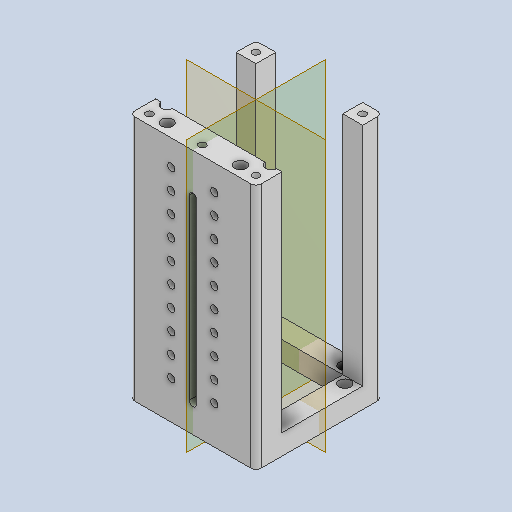
# Autodesk Inventor part: 00_Linear_Stage_NEMA11_Mount
Saved by Autodesk Inventor 2023 (Build 270158000, 158)
## iProperties
Created: 2022-02-11
Part Number: 00_Linear_Stage_NEMA11_Mount
Material: Generic
Document SubType Name: Modeling
Designer: wanghaoran
Density: 1 g/cm^3
Appearance: Default
Author: wanghaoran
Autodesk Inventor part; units mm, degrees
ref_plane "YZ Plane" through (0, 0, 0) normal (1, 0, 0) x (0, 1, 0)
ref_plane "XZ Plane" through (0, 0, 0) normal (0, 1, 0) x (-1, 0, 0)
ref_plane "XY Plane" through (0, 0, 0) normal (0, 0, 1) x (1, 0, 0)
sketch "Sketch1" plane through (0, 0, 0) normal (0, 1, 0) x (-1, 0, 0)
  line L0 (0, 0) -> (49.8, 0)
  line L1 (49.8, 0) -> (49.8, -49.8)
  line L2 (49.8, -49.8) -> (0, -49.8)
  line L3 (0, -49.8) -> (0, 0)
  line L4 (7.8, -7.8) -> (42, -7.8)
  line L5 (42, -7.8) -> (42, -42)
  line L6 (42, -42) -> (7.8, -42)
  line L7 (7.8, -42) -> (7.8, -7.8)
  dimension "d0" = 49.8
  dimension "d1" = 49.8
  dimension "d2" = 7.8
  constraints: 16 end point, 4 parallel, 2 perpendicular, 1 horizontal, 3 other
  measures "d0" distance of L1.end L2.end
  measures "d1" distance of L0.end L1.end
  measures "d2" distance between parallel lines of L3 L7
extrude "Extrusion1" add sketch "Sketch1" along normal blind 8
sketch "Sketch3" plane through (0, 0, 0) normal (0, -1, 0) x (1, 0, 0)
  line L0 (-49.8, 0) -> (0, 0) projected
  line L1 (-49.8, -49.8) -> (-49.8, 0) projected
  line L2 (0, 0) -> (-49.8, 0)
  line L3 (-49.8, 0) -> (-49.8, -10.23)
  line L4 (-49.8, -10.23) -> (0, -10.23)
  line L5 (0, -10.23) -> (0, 0)
  line L6 (-7.8, -42) -> (-7.8, -7.8) projected
  line L7 (0, -49.8) -> (-7.8, -49.8)
  line L8 (-7.8, -49.8) -> (-7.8, -42)
  line L9 (-7.8, -42) -> (0, -42)
  line L10 (0, -42) -> (0, -49.8)
  line L11 (0, -49.8) -> (-49.8, -49.8) projected
  line L12 (-42, -7.8) -> (-42, -42) projected
  line L13 (-49.8, -49.8) -> (-42, -49.8)
  line L14 (-42, -49.8) -> (-42, -42)
  line L15 (-42, -42) -> (-49.8, -42)
  line L16 (-49.8, -42) -> (-49.8, -49.8)
  dimension "d6" = 10.23
  constraints: 24 end point, 6 parallel, 3 horizontal, 3 perpendicular, 1 point on line
  measures "d6" distance of L3.end L2.end
extrude "Extrusion2" add sketch "Sketch3" against normal blind 97 contours L0 L5 L4 L1 | L15 L14 L11 L1 | L9 L10 L7 L8
sketch "Sketch4" plane through (-49.8, 0, 0) normal (0, 0, 1) x (1, 0, 0)
  line L0 (23.45, 81) -> (26.35, 81)
  line L1 (26.35, 81) -> (26.35, 11)
  line L2 (26.35, 11) -> (23.45, 11)
  line L3 (23.45, 11) -> (23.45, 81)
  line L4 (49.8, 0) -> (49.8, 97) projected
  line L5 (0, 0) -> (49.8, 0) projected
  circle A0 centre (24.9, 81) radius 1.45
  circle A1 centre (24.9, 11) radius 1.45
  circle A2 centre (16.4, 87) radius 1.45
  circle A3 centre (33.4, 87) radius 1.45
  line L6 (0, 97) -> (49.8, 97) projected
  circle A4 centre (16.4, 79) radius 1.45
  circle A5 centre (33.4, 79) radius 1.45
  circle A6 centre (16.4, 71) radius 1.45
  circle A7 centre (33.4, 71) radius 1.45
  circle A8 centre (16.4, 63) radius 1.45
  circle A9 centre (33.4, 63) radius 1.45
  circle A10 centre (16.4, 55) radius 1.45
  circle A11 centre (33.4, 55) radius 1.45
  circle A12 centre (16.4, 47) radius 1.45
  circle A13 centre (33.4, 47) radius 1.45
  circle A14 centre (16.4, 39) radius 1.45
  circle A15 centre (33.4, 39) radius 1.45
  circle A16 centre (16.4, 31) radius 1.45
  circle A17 centre (33.4, 31) radius 1.45
  circle A18 centre (16.4, 23) radius 1.45
  circle A19 centre (33.4, 23) radius 1.45
  circle A20 centre (16.4, 15) radius 1.45
  circle A21 centre (33.4, 15) radius 1.45
  point P0 (32.35, 97)
  point P1 (34.45, 97)
  dimension "d9" = 2.9
  dimension "d10" = 70
  dimension "d11" = 23.45
  dimension "d12" = 11
  dimension "d15" = 2.9
  dimension "d16" = 7.05
  dimension "d17" = 2.9
  dimension "d18" = 7.05
  dimension "d19" = 10
  dimension "d20" = 10
  dimension "d23" = 8
  dimension "d52" = 8
  constraints: 20 centre point, 8 end point, 2 midpoint, 2 parallel, 2 vertical, 1 horizontal, 1 perpendicular, 42 other
  measures "d9" distance of L1.end L2.end
  measures "d10" distance of L0.end L1.end
  measures "d11" distance between parallel lines of L4 L1
  measures "d12" distance between parallel lines of L5 L2
  measures "d15" diameter of A2
  measures "d16" distance from line of L3 A2.centre
  measures "d17" diameter of A3
  measures "d18" distance from line of A3.centre L1
  measures "d19" distance from line of L6 A2.centre
  measures "d20" distance from line of L6 A3.centre
  measures "d23" distance of A2.centre A4.centre
  measures "d52" distance of A14.centre A16.centre
extrude "Extrusion3" cut sketch "Sketch4" against normal through all
sketch "Sketch5" plane through (0, 97, 0) normal (0, 1, 0) x (1, 0, 0)
  circle A0 centre (-45.9, 45.9) radius 1.4
  circle A1 centre (-3.9, 45.9) radius 1.4
  line L0 (-49.8, 49.8) -> (-49.8, 0) projected
  line L1 (-49.8, 24.9) -> (-42, 24.9)
  line L2 (-42, 10.23) -> (-42, 42) projected
  circle A2 centre (-45.9, 3.9) radius 1.4
  circle A3 centre (-3.9, 3.9) radius 1.4
  point P0 (0, 0)
  dimension "d28" = 2.8
  dimension "d29" = 2.8
  constraints: 4 centre point, 2 end point, 2 symmetric about line, 1 horizontal, 1 midpoint, 1 point on line, 2 other
  measures "d28" diameter of A0
  measures "d29" diameter of A1
extrude "Extrusion4" cut sketch "Sketch5" against normal blind 20
sketch "Sketch6" plane through (0, 0, 0) normal (0, -1, 0) x (1, 0, 0)
  line L0 (-49.8, 0) -> (0, 0) projected
  circle A0 centre (-24.9, -3.7) radius 1.4
  line L1 (-49.8, -49.8) -> (-49.8, 0) projected
  dimension "d37" = 2.8
  dimension "d38" = 3.7
  dimension "d39" = 24.9
  constraints: 1 centre point
  measures "d37" diameter of A0
  measures "d38" distance from line of L0 A0.centre
  measures "d39" distance from line of L1 A0.centre
extrude "Extrusion5" cut sketch "Sketch6" against normal blind 10
fillet "Fillet1" radius 2 4 edges at (0, 48.5, 0) (0, 48.5, -49.8) (-49.8, 48.5, -49.8) (-49.8, 48.5, 0)
sketch "Sketch7" plane through (0, 97, 0) normal (0, 1, 0) x (1, 0, 0)
  circle A0 centre (-24.9, 3.7) radius 1.4 projected
  circle A1 centre (-24.9, 3.7) radius 1.4
  point P0 (0, 0)
  constraints: 1 centre point, 1 coincident
extrude "Extrusion6" cut sketch "Sketch7" against normal blind 10
ref_plane "Arbeitsebene1" through (-24.9, 8, -10.23) normal (-1, 0, 0) x (0, 0, 1)
ref_plane "Arbeitsebene2" through (-47.8, 0, -24.9) normal (0, 0, 1) x (1, 0, 0)
sketch "Skizze8" plane through (0, 0, 0) normal (0, -1, 0) x (1, 0, 0)
  line L0 (-49.9, -29.9) -> (-49.9, -47.9) projected
  arc A0 (-49.9, -47.9) -> (-47.9, -49.9) centre (-47.9, -47.9) ccw projected
  line L1 (-30.0511, -49.9) -> (-47.9, -49.9) projected
  line L2 (-30.0511, -49.9) -> (-30.0509, -49.1742) projected
  arc A1 (-30.0509, -49.1742) -> (-30.2806, -48.8498) centre (-30.3999, -49.1778) ccw projected
  arc A2 (-31.9947, -46.7407) -> (-30.2806, -48.8498) centre (-29.84, -46.7407) ccw projected
  line L3 (-31.9947, -46.7407) -> (-31.9947, -46.6009) projected
  arc A3 (-29.8434, -44.4498) -> (-31.9947, -46.6009) centre (-29.8435, -46.6009) ccw projected
  line L4 (-29.8434, -44.4498) -> (-19.9598, -44.4503) projected
  arc A4 (-17.81, -46.6004) -> (-19.9598, -44.4503) centre (-19.96, -46.6003) ccw projected
  line L5 (-17.81, -46.6004) -> (-17.81, -46.7408) projected
  arc A5 (-19.52, -48.8451) -> (-17.81, -46.7408) centre (-19.9599, -46.7406) ccw projected
  arc A6 (-19.52, -48.8451) -> (-19.7498, -49.1739) centre (-19.3996, -49.1739) ccw projected
  line L6 (-19.7498, -49.1739) -> (-19.7495, -49.9) projected
  line L7 (-1.9, -49.9) -> (-19.7495, -49.9) projected
  arc A7 (-1.9, -49.9) -> (0.1, -47.9) centre (-1.9, -47.9) ccw projected
  line L8 (0.1, -47.9) -> (0.1, -30.0511) projected
  line L9 (0.1, -30.0511) -> (-0.6258, -30.0509) projected
  arc A8 (-0.6258, -30.0509) -> (-0.9502, -30.2806) centre (-0.6222, -30.3999) ccw projected
  arc A9 (-3.0593, -31.9947) -> (-0.9502, -30.2806) centre (-3.0593, -29.84) ccw projected
  line L10 (-3.0593, -31.9947) -> (-3.1991, -31.9947) projected
  arc A10 (-5.3502, -29.8434) -> (-3.1991, -31.9947) centre (-3.1991, -29.8435) ccw projected
  line L11 (-5.3502, -29.8434) -> (-5.3497, -19.9598) projected
  arc A11 (-3.1996, -17.81) -> (-5.3497, -19.9598) centre (-3.1997, -19.96) ccw projected
  line L12 (-3.1996, -17.81) -> (-3.0592, -17.81) projected
  arc A12 (-0.9549, -19.52) -> (-3.0592, -17.81) centre (-3.0594, -19.9599) ccw projected
  arc A13 (-0.9549, -19.52) -> (-0.6261, -19.7498) centre (-0.6261, -19.3996) ccw projected
  line L13 (-0.6261, -19.7498) -> (0.1, -19.7495) projected
  line L14 (0.1, -19.7495) -> (0.1, -1.9) projected
  arc A14 (0.1, -1.9) -> (-1.9, 0.1) centre (-1.9, -1.9) ccw projected
  line L15 (-19.9, 0.1) -> (-1.9, 0.1) projected
  line L16 (-19.9, 0.1) -> (-19.9, 0.9263) projected
  arc A15 (-19.56, 1.4) -> (-19.9, 0.9263) centre (-19.4, 0.9263) ccw projected
  arc A16 (-19.56, 1.4) -> (-17.96, 3.3596) centre (-19.96, 3.3596) ccw projected
  line L17 (-17.96, 3.3596) -> (-17.96, 3.5) projected
  arc A17 (-17.96, 3.5) -> (-19.96, 5.5) centre (-19.96, 3.5) ccw projected
  line L18 (-19.96, 5.5) -> (-29.84, 5.5) projected
  arc A18 (-29.84, 5.5) -> (-31.84, 3.5) centre (-29.84, 3.5) ccw projected
  line L19 (-31.84, 3.5) -> (-31.84, 3.3596) projected
  arc A19 (-31.84, 3.3596) -> (-30.24, 1.4) centre (-29.84, 3.3596) ccw projected
  arc A20 (-29.9, 0.9263) -> (-30.24, 1.4) centre (-30.4, 0.9263) ccw projected
  line L20 (-29.9, 0.9263) -> (-29.9, 0.1) projected
  line L21 (-47.9, 0.1) -> (-29.9, 0.1) projected
  arc A21 (-47.9, 0.1) -> (-49.9, -1.9) centre (-47.9, -1.9) ccw projected
  line L22 (-49.9, -1.9) -> (-49.9, -19.9) projected
  line L23 (-49.9, -19.9) -> (-50.7263, -19.9) projected
  arc A22 (-51.2, -19.56) -> (-50.7263, -19.9) centre (-50.7263, -19.4) ccw projected
  arc A23 (-51.2, -19.56) -> (-53.1596, -17.96) centre (-53.1596, -19.96) ccw projected
  line L24 (-53.1596, -17.96) -> (-53.3, -17.96) projected
  arc A24 (-53.3, -17.96) -> (-55.3, -19.96) centre (-53.3, -19.96) ccw projected
  line L25 (-55.3, -19.96) -> (-55.3, -29.84) projected
  arc A25 (-55.3, -29.84) -> (-53.3, -31.84) centre (-53.3, -29.84) ccw projected
  line L26 (-53.3, -31.84) -> (-53.1596, -31.84) projected
  arc A26 (-53.1596, -31.84) -> (-51.2, -30.24) centre (-53.1596, -29.84) ccw projected
  arc A27 (-50.7263, -29.9) -> (-51.2, -30.24) centre (-50.7263, -30.4) ccw projected
  line L27 (-50.7263, -29.9) -> (-49.9, -29.9) projected
  arc A28 (-49.9, -26.2329) -> (-49.9, -23.7671) centre (-46.2, -25) ccw projected
  line L28 (-49.9, -26.2329) -> (-49.9, -23.7671) projected
  circle A29 centre (-25, -3.6) radius 3.9 projected
  line L29 (-7.6, -40.2) -> (-7.6, -9.6) projected
  arc A30 (-9.6, -42.2) -> (-7.6, -40.2) centre (-9.6, -40.2) ccw projected
  line L30 (-9.6, -42.2) -> (-40.2, -42.2) projected
  arc A31 (-42.2, -40.2) -> (-40.2, -42.2) centre (-40.2, -40.2) ccw projected
  line L31 (-42.2, -9.6) -> (-42.2, -40.2) projected
  arc A32 (-40.2, -7.6) -> (-42.2, -9.6) centre (-40.2, -9.6) ccw projected
  line L32 (-40.2, -7.6) -> (-9.6, -7.6) projected
  arc A33 (-7.6, -9.6) -> (-9.6, -7.6) centre (-9.6, -9.6) ccw projected
  circle A34 centre (-44.8, -5) radius 2.4 projected
  circle A35 centre (-39.35, -4.35) radius 2.45 projected
  circle A36 centre (-45.45, -10.45) radius 2.45 projected
  circle A37 centre (-4.35, -10.45) radius 2.45 projected
  circle A38 centre (-10.45, -4.35) radius 2.45 projected
  circle A39 centre (-5, -5) radius 2.4 projected
  circle A40 centre (-45.45, -39.35) radius 2.45 projected
  circle A41 centre (-39.35, -45.45) radius 2.45 projected
  circle A42 centre (-44.8, -44.8) radius 2.4 projected
  circle A43 centre (-4.35, -39.35) radius 2.45 projected
  circle A44 centre (-10.45, -45.45) radius 2.45 projected
  circle A45 centre (-5, -44.8) radius 2.4 projected
  point P0 (0, 0)
hole "Bohrung1" at (-45.45, 0, -39.35) at (-45.45, 0, -10.45) at (-39.35, 0, -4.35) at (-10.45, 0, -4.35) at (-4.35, 0, -10.45) at (-4.35, 0, -39.35) at (-10.45, 0, -45.45) at (-39.35, 0, -45.45) direction (0, 1, 0) diameter 4.6 end through all
body "Solid1"
